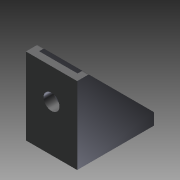
# Autodesk Inventor part: HBLFSNE6_
Saved by Autodesk Inventor 2011 SP1 (Build 150282100, 282)
## iProperties
Created: 2016-11-23
Part Number: HBLFSNE6_
Catalog Web Link: www.cadenas.de
Description: HBLFSN6, HBLFSNB6, HBLFSNM6, HBLFSNK6, HBLFSSW6, HBLFSSWB6, HBLFSSW6-50, HBLFSDW6, HBLFSDW6-50, HBLFSN6, HBLFSD6-50-Thin Reversal Brackets for Slot Width 8 Frames - For 30, 50, 60mm Sections
Vendor: MISUMI
Document SubType Name: Modeling
Designer: psAdmin
Manufacturer: MISUMI
Mass: 6.00076 g
Surface Area: 42.7763 cm^2
Volume: 6.00076 cm^3
Density: 1 g/cm^3
Category: PARTsolutions
Company: MISUMI
Title: HBLFSNE6_
Author: Cadenas PARTsolutions
Comments: Thin Reversal Brackets for Slot Width 8 Frames - For 30, 50, 60mm Sections
PSOL_IDENT_0: {$CADENAS_DATA\23d-libs\misumi\metric\38_al_extrusions_blackets\6\hblfsn6.prj},279 {VTYP=3D},{NB=HBL
PSOL_IDENT_1: FSNE6_},{LINA=HBLFSNE6_},{NN=HBLFSN6, HBLFSNB6, HBLFSNM6, HBLFSNK6, HBLFSSW6, HBLFSSWB6, HBLFSSW6-50
PSOL_IDENT_2: , HBLFSDW6, HBLFSDW6-50, HBLFSN6, HBLFSD6-50},{DATE=17.06.2016 05:53:15},{GEOMDATE=09.11.2010 09:07:
PSOL_IDENT_3: 00},{VERSION=},{LINEID=350},{LINESUBID=-1},{WBVAR=ALT1,ALT2}  {NB=HBLFSNE6_},{LINA=HBLFSNE6_},{KT=1}
PSOL_IDENT_4: ,{PN=HBLFSNE6},{TP=HBLFSNE6},{NOH=1},{NOHV=1},{MAT=ADC12},{ST=-},{TYPE=HBLFSNE6},{FEAT=Bracket with
PSOL_IDENT_5: Single Side Protrusion},{ALT1=},{ALT2=},{MASS=15},{AB=CBM6-12},{NOB=2},{AN=HNTT6-6},{NON=2},{AL=1176
PSOL_IDENT_6: },{W=20},{H=30},{DP=30},{T=4.5},{HDIS=8},{DPOS=12},{HH1=18},{HV1=15},{DIA=6.2},{ALT1OPT='','w/o C (M
PSOL_IDENT_7: ounting Holes for Cover)','-C','with C (Mounting Holes for Cover)'},{ALT2OPT= '' , 'w/o Set Applicab
PSOL_IDENT_8: le Bolt & Nut' , '-SET' , 'with SET (Set Applicable Bolt & Nut)' , '-SST' , 'with SST (Stainless Ste
PSOL_IDENT_9: el Set Applicable Bolt & Nut)' , '-SEP' , 'with SEP (Post Assembly Spring Nuts Set Applicable Bolt &
PSOL_IDENT_10: Nut)' , '-SSP' , 'with SSP (Post Assembly Spring Nuts, Stainless Steel Set Applicable Bolt & Nut)'}
PSOL_IDENT_11: ,{R=1},{R1=0.3},{APOSV=0},{VER=1},{PR=1},{TT=1.0},{T1=2}
NN: HBLFSN6, HBLFSNB6, HBLFSNM6, HBLFSNK6, HBLFSSW6, HBLFSSWB6, HBLFSSW6-50, HBLFSDW6, HBLFSDW6-50, HBLFSN6, HBLFSD6-50
NT: Thin Reversal Brackets for Slot Width 8 Frames - For 30, 50, 60mm Sections
NB: HBLFSNE6_
NBSYN: $PN._
LINA: HBLFSNE6_
PN: HBLFSNE6
TP: HBLFSNE6
MAT: ADC12
ST: -
FEAT: Bracket with Single Side Protrusion
ALT1: w/o C (Mounting Holes for Cover)
ALT2: w/o Set Applicable Bolt & Nut
MASS: 15
AB: CBM6-12
NOB: 2
AN: HNTT6-6
NON: 2
AL: 1176
SUPPLIER: MISUMI
ARTICLENO: HBLFSNE6_
BOMINFO: HBLFSNE6_
CREATOR: CADENAS GmbH
Autodesk Inventor part; units mm, degrees
sketch "Sketch_15" plane through (0, 0, 0) normal (1, 0, 0) x (0, 1, 0)
  line L0 (0, 30) -> (0, 0)
  line L1 (0, 0) -> (30, 0)
  line L2 (30, 0) -> (30, 4.0858)
  arc A0 (30, 4.0858) -> (29.7071, 4.7929) centre (29, 4.0858) ccw
  line L3 (29.7071, 4.7929) -> (4.7929, 29.7071)
  arc A1 (4.7929, 29.7071) -> (4.0858, 30) centre (4.0858, 29) ccw
  line L4 (4.0858, 30) -> (0, 30)
  constraints: 10 end point, 4 point on circle, 2 centre point
extrude "Extrusion1" add sketch "Sketch_15" along normal mid plane 20
sketch "Sketch_16" plane through (0, 0, 0) normal (1, 0, 0) x (0, 1, 0)
  line L0 (2.9278, 34.5) -> (4.4738, 5)
  line L1 (4.4738, 5) -> (34.5, 5)
  line L2 (34.5, 5) -> (34.5, 34.5)
  line L3 (34.5, 34.5) -> (2.9278, 34.5)
  constraints: 8 end point
extrude "Extrusion2" cut sketch "Sketch_16" along normal mid plane 15
sketch "Sketch_82" plane through (0, 0, 0) normal (1, 0, 0) x (0, 1, 0)
  line L0 (2.4278, 34.5) -> (4, 4.5)
  line L1 (4, 4.5) -> (34, 4.5)
  line L2 (34, 4.5) -> (34, 34.5)
  line L3 (34, 34.5) -> (2.4278, 34.5)
  constraints: 8 end point
extrude "Extrusion3" cut sketch "Sketch_82" along normal mid plane 15
sketch "Sketch_17" plane through (0, 4.5, 0) normal (0, 1, 0) x (1, 0, 0)
  line L0 (-5.4209, -10.5) -> (-4.4687, -18.5299)
  arc A0 (-4.4687, -18.5299) -> (4.4687, -18.5299) centre (0, -18) ccw
  line L1 (4.4687, -18.5299) -> (5.4209, -10.5)
  line L2 (5.4209, -10.5) -> (-5.4209, -10.5)
  constraints: 6 end point, 2 point on circle, 1 centre point
extrude "Extrusion4" add sketch "Sketch_17" against normal blind 2.25
sketch "Sketch5" plane through (10, 0, 0) normal (0, 0, -1) x (-1, 0, 0)
  point P0 (10, 15)
hole "Hole1" at (0, 15, 0) direction (0, 0, 1) diameter 6.2 depth 5.5
sketch "Sketch6" plane through (-10, 0, 30) normal (0, -1, 0) x (1, 0, 0)
  point P0 (10, -12)
hole "Hole2" at (0, 0, 18) direction (0, 1, 0) diameter 6.2 depth 4.5
sketch "Sketch_1" plane through (0, 0, 0) normal (0, 1, 0) x (-1, 0, 0)
  line L0 (10, 0) -> (10, 30)
  line L1 (10, 30) -> (-10, 30)
  line L2 (-10, 30) -> (-10, 0)
  line L3 (-10, 0) -> (10, 0)
  constraints: 8 end point
extrude "Extrusion5" add sketch "Sketch_1" against normal blind 1
sketch "Sketch_4" plane through (0, 0, 0) normal (0, 1, 0) x (-1, 0, 0)
  line L0 (10, 0) -> (10, 30)
  line L1 (10, 30) -> (-10, 30)
  line L2 (-10, 30) -> (-10, 0)
  line L3 (-10, 0) -> (10, 0)
  constraints: 8 end point
extrude "Extrusion6" cut sketch "Sketch_4" against normal blind 1
sketch "Sketch_72" plane through (0, 0, 0) normal (0, 0, 1) x (1, 0, 0)
  line L0 (-3.6, 14.5) -> (-3.6, 11.6)
  arc A0 (-3.6, 11.6) -> (-3.4, 11.4) centre (-3.4, 11.6) ccw
  line L1 (-3.4, 11.4) -> (3.4, 11.4)
  arc A1 (3.4, 11.4) -> (3.6, 11.6) centre (3.4, 11.6) ccw
  line L2 (3.6, 11.6) -> (3.6, 14.5)
  line L3 (3.6, 14.5) -> (3.0594, 14.5)
  arc A2 (-3.0594, 14.5) -> (3.0594, 14.5) centre (0, 15) ccw
  line L4 (-3.0594, 14.5) -> (-3.6, 14.5)
  constraints: 10 end point, 6 point on circle, 3 centre point
extrude "Extrusion7" add sketch "Sketch_72" against normal blind 1
sketch "Sketch_73" plane through (0, 0, 0) normal (0, 0, 1) x (1, 0, 0)
  line L0 (-3.6, 15.5) -> (-3.0594, 15.5)
  arc A0 (3.0594, 15.5) -> (-3.0594, 15.5) centre (0, 15) ccw
  line L1 (3.0594, 15.5) -> (3.6, 15.5)
  line L2 (3.6, 15.5) -> (3.6, 18.4)
  arc A1 (3.6, 18.4) -> (3.4, 18.6) centre (3.4, 18.4) ccw
  line L3 (3.4, 18.6) -> (-3.4, 18.6)
  arc A2 (-3.4, 18.6) -> (-3.6, 18.4) centre (-3.4, 18.4) ccw
  line L4 (-3.6, 18.4) -> (-3.6, 15.5)
  constraints: 10 end point, 6 point on circle, 3 centre point
extrude "Extrusion8" add sketch "Sketch_73" against normal blind 1
sketch "Sketch_86" plane through (0, 4.5, 0) normal (0, 1, 0) x (1, 0, 0)
  line L0 (-5.4209, -10.5) -> (-4.4687, -18.5299)
  arc A0 (-4.4687, -18.5299) -> (4.4687, -18.5299) centre (0, -18) ccw
  line L1 (4.4687, -18.5299) -> (5.4209, -10.5)
  line L2 (5.4209, -10.5) -> (-5.4209, -10.5)
  constraints: 6 end point, 2 point on circle, 1 centre point
extrude "Extrusion9" cut sketch "Sketch_86" against normal blind 0.5
ref_plane "SD6_50_1_XY" through (-10, 15, 4.5) normal (0, 0, 1) x (1, 0, 0)
ref_plane "SD6_50_1_YZ" through (-10, 15, 4.5) normal (1, 0, 0) x (0, 1, 0)
ref_plane "SD6_50_1_ZX" through (-10, 15, 4.5) normal (0, 1, 0) x (0, 0, 1)
ref_plane "SD6_50_2_XY" through (10, 15, 4.5) normal (0, 0, 1) x (1, 0, 0)
ref_plane "SD6_50_2_YZ" through (10, 15, 4.5) normal (1, 0, 0) x (0, 1, 0)
ref_plane "SD6_50_2_ZX" through (10, 15, 4.5) normal (0, 1, 0) x (0, 0, 1)
ref_plane "SD6_50_3_XY" through (-10, 4.5, 18) normal (0, 1, 0) x (1, 0, 0)
ref_plane "SD6_50_3_YZ" through (-10, 4.5, 18) normal (1, 0, 0) x (0, 0, -1)
ref_plane "SD6_50_3_ZX" through (-10, 4.5, 18) normal (0, 0, -1) x (0, 1, 0)
ref_plane "SD6_50_4_XY" through (10, 4.5, 18) normal (0, 1, 0) x (1, 0, 0)
ref_plane "SD6_50_4_YZ" through (10, 4.5, 18) normal (1, 0, 0) x (0, 0, -1)
ref_plane "SD6_50_4_ZX" through (10, 4.5, 18) normal (0, 0, -1) x (0, 1, 0)
ref_plane "a10_to_bolt_XY" through (15, 15, 4.5) normal (0, 0, 1) x (1, 0, 0)
ref_plane "a10_to_bolt_YZ" through (15, 15, 4.5) normal (1, 0, 0) x (0, 1, 0)
ref_plane "a10_to_bolt_ZX" through (15, 15, 4.5) normal (0, 1, 0) x (0, 0, 1)
ref_plane "a11_to_bolt_XY" through (-15, 4.5, 18) normal (0, 1, 0) x (1, 0, 0)
ref_plane "a11_to_bolt_YZ" through (-15, 4.5, 18) normal (1, 0, 0) x (0, 0, -1)
ref_plane "a11_to_bolt_ZX" through (-15, 4.5, 18) normal (0, 0, -1) x (0, 1, 0)
ref_plane "a12_to_bolt_XY" through (15, 4.5, 18) normal (0, 1, 0) x (1, 0, 0)
ref_plane "a12_to_bolt_YZ" through (15, 4.5, 18) normal (1, 0, 0) x (0, 0, -1)
ref_plane "a12_to_bolt_ZX" through (15, 4.5, 18) normal (0, 0, -1) x (0, 1, 0)
ref_plane "a13_to_bolt_XY" through (0, 4.5, 38) normal (0, 1, 0) x (1, 0, 0)
ref_plane "a13_to_bolt_YZ" through (0, 4.5, 38) normal (1, 0, 0) x (0, 0, -1)
ref_plane "a13_to_bolt_ZX" through (0, 4.5, 38) normal (0, 0, -1) x (0, 1, 0)
ref_plane "a14_to_bolt_XY" through (0, 30, 4.5) normal (0, 0, 1) x (1, 0, 0)
ref_plane "a14_to_bolt_YZ" through (0, 30, 4.5) normal (1, 0, 0) x (0, 1, 0)
ref_plane "a14_to_bolt_ZX" through (0, 30, 4.5) normal (0, 1, 0) x (0, 0, 1)
ref_plane "a1_to_bolt_XY" through (-10, 20, 4.5) normal (0, 0, 1) x (1, 0, 0)
ref_plane "a1_to_bolt_YZ" through (-10, 20, 4.5) normal (1, 0, 0) x (0, 1, 0)
ref_plane "a1_to_bolt_ZX" through (-10, 20, 4.5) normal (0, 1, 0) x (0, 0, 1)
ref_plane "a2_to_bolt_XY" through (-10, 4.5, 15) normal (0, 1, 0) x (1, 0, 0)
ref_plane "a2_to_bolt_YZ" through (-10, 4.5, 15) normal (1, 0, 0) x (0, 0, -1)
ref_plane "a2_to_bolt_ZX" through (-10, 4.5, 15) normal (0, 0, -1) x (0, 1, 0)
ref_plane "a3_to_bolt_XY" through (1, 15, 4.5) normal (0, 0, 1) x (1, 0, 0)
ref_plane "a3_to_bolt_YZ" through (1, 15, 4.5) normal (1, 0, 0) x (0, 1, 0)
ref_plane "a3_to_bolt_ZX" through (1, 15, 4.5) normal (0, 1, 0) x (0, 0, 1)
ref_plane "a4_to_bolt_XY" through (1, 4, 18) normal (0, 1, 0) x (1, 0, 0)
ref_plane "a4_to_bolt_YZ" through (1, 4, 18) normal (1, 0, 0) x (0, 0, -1)
ref_plane "a4_to_bolt_ZX" through (1, 4, 18) normal (0, 0, -1) x (0, 1, 0)
ref_plane "a55_to_bolt_XY" through (0, 18, 4.5) normal (0, 0, 1) x (1, 0, 0)
ref_plane "a55_to_bolt_YZ" through (0, 18, 4.5) normal (1, 0, 0) x (0, 1, 0)
ref_plane "a55_to_bolt_ZX" through (0, 18, 4.5) normal (0, 1, 0) x (0, 0, 1)
ref_plane "a5_to_bolt_XY" through (0, 15, 4.5) normal (0, 0, 1) x (1, 0, 0)
ref_plane "a5_to_bolt_YZ" through (0, 15, 4.5) normal (1, 0, 0) x (0, 1, 0)
ref_plane "a5_to_bolt_ZX" through (0, 15, 4.5) normal (0, 1, 0) x (0, 0, 1)
ref_plane "a6_to_bolt_XY" through (0, 4, 18) normal (0, 1, 0) x (1, 0, 0)
ref_plane "a6_to_bolt_YZ" through (0, 4, 18) normal (1, 0, 0) x (0, 0, -1)
ref_plane "a6_to_bolt_ZX" through (0, 4, 18) normal (0, 0, -1) x (0, 1, 0)
ref_plane "a7_to_bolt_XY" through (0, 35, 4.5) normal (0, 0, 1) x (1, 0, 0)
ref_plane "a7_to_bolt_YZ" through (0, 35, 4.5) normal (1, 0, 0) x (0, 1, 0)
ref_plane "a7_to_bolt_ZX" through (0, 35, 4.5) normal (0, 1, 0) x (0, 0, 1)
ref_plane "a8_to_bolt_XY" through (0, 4.5, 48) normal (0, 1, 0) x (1, 0, 0)
ref_plane "a8_to_bolt_YZ" through (0, 4.5, 48) normal (1, 0, 0) x (0, 0, -1)
ref_plane "a8_to_bolt_ZX" through (0, 4.5, 48) normal (0, 0, -1) x (0, 1, 0)
ref_plane "a9_to_bolt_XY" through (-15, 15, 4.5) normal (0, 0, 1) x (1, 0, 0)
ref_plane "a9_to_bolt_YZ" through (-15, 15, 4.5) normal (1, 0, 0) x (0, 1, 0)
ref_plane "a9_to_bolt_ZX" through (-15, 15, 4.5) normal (0, 1, 0) x (0, 0, 1)
ref_plane "bracket_to_dummy_XY" through (0, 0, 0) normal (0, 1, 0) x (1, 0, 0)
ref_plane "bracket_to_dummy_YZ" through (0, 0, 0) normal (1, 0, 0) x (0, 0, -1)
ref_plane "bracket_to_dummy_ZX" through (0, 0, 0) normal (0, 0, -1) x (0, 1, 0)
ref_plane "hole_x1_bolt_XY" through (-10, 35, 4.5) normal (0, 0, 1) x (1, 0, 0)
ref_plane "hole_x1_bolt_YZ" through (-10, 35, 4.5) normal (1, 0, 0) x (0, 1, 0)
ref_plane "hole_x1_bolt_ZX" through (-10, 35, 4.5) normal (0, 1, 0) x (0, 0, 1)
ref_plane "holex2_to_bolt_XY" through (10, 35, 4.5) normal (0, 0, 1) x (1, 0, 0)
ref_plane "holex2_to_bolt_YZ" through (10, 35, 4.5) normal (1, 0, 0) x (0, 1, 0)
ref_plane "holex2_to_bolt_ZX" through (10, 35, 4.5) normal (0, 1, 0) x (0, 0, 1)
ref_plane "holex3_to_bolt_XY" through (10, 4.5, 35) normal (0, 1, 0) x (1, 0, 0)
ref_plane "holex3_to_bolt_YZ" through (10, 4.5, 35) normal (1, 0, 0) x (0, 0, -1)
ref_plane "holex3_to_bolt_ZX" through (10, 4.5, 35) normal (0, 0, -1) x (0, 1, 0)
ref_plane "holex4_to_bolt_XY" through (10, 4.5, 15) normal (0, 1, 0) x (1, 0, 0)
ref_plane "holex4_to_bolt_YZ" through (10, 4.5, 15) normal (1, 0, 0) x (0, 0, -1)
ref_plane "holex4_to_bolt_ZX" through (10, 4.5, 15) normal (0, 0, -1) x (0, 1, 0)
ref_plane "holex5_to_bolt_XY" through (-10, 4.5, 35) normal (0, 1, 0) x (1, 0, 0)
ref_plane "holex5_to_bolt_YZ" through (-10, 4.5, 35) normal (1, 0, 0) x (0, 0, -1)
ref_plane "holex5_to_bolt_ZX" through (-10, 4.5, 35) normal (0, 0, -1) x (0, 1, 0)
ref_plane "holex6_to_bolt_XY" through (10, 20, 4.5) normal (0, 0, 1) x (1, 0, 0)
ref_plane "holex6_to_bolt_YZ" through (10, 20, 4.5) normal (1, 0, 0) x (0, 1, 0)
ref_plane "holex6_to_bolt_ZX" through (10, 20, 4.5) normal (0, 1, 0) x (0, 0, 1)
body "Solid1"
